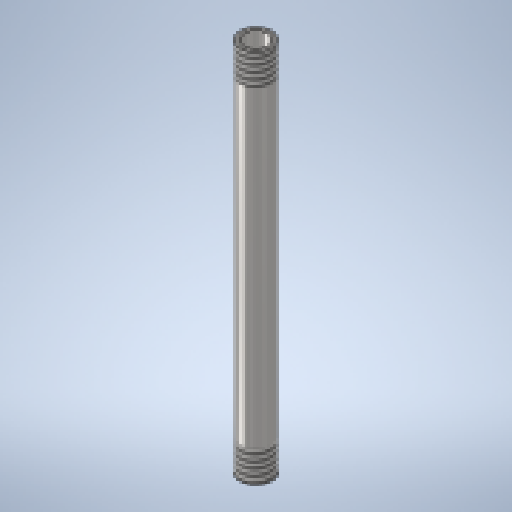
# Autodesk Inventor part: Shaft - Flywheel
Saved by Autodesk Inventor 2023.2 (Build 272271000, 271)
## iProperties
Created: 2024-02-13
Part Number: Shaft - Flywheel
Material: Steel, Alloy
Document SubType Name: Modeling
Designer: Nathan Cai
Mass: 8.98376 g
Surface Area: 26.4511 cm^2
Volume: 1.16219 cm^3
Density: 7.73 g/cm^3
Appearance: Semi-Polished
Author: Nathan Cai
Autodesk Inventor part; units mm, degrees
ref_plane "YZ Plane" through (0, 0, 0) normal (1, 0, 0) x (0, 1, 0)
ref_plane "XZ Plane" through (0, 0, 0) normal (0, 1, 0) x (-1, 0, 0)
ref_plane "XY Plane" through (0, 0, 0) normal (0, 0, 1) x (1, 0, 0)
sketch "Sketch1" plane through (0, 0, 0) normal (0, 1, 0) x (-1, 0, 0)
  circle A0 centre (0, 0) radius 3.175
  circle A1 centre (0, 0) radius 2.286
  dimension "d0" = 6.35
  dimension "d1" = 4.572
  constraints: 2 centre point, 2 coincident
  measures "d0" diameter of A0
  measures "d1" diameter of A1
extrude "Extrusion1" add sketch "Sketch1" along normal blind 76.2
thread "Thread1" size "1/4-20 UNC" class "2A" standard "ANSI Unified Screw Threads" length 6.35
thread "Thread2" size "1/4-20 UNC" class "2A" standard "ANSI Unified Screw Threads" length 6.35
body "Solid1"
